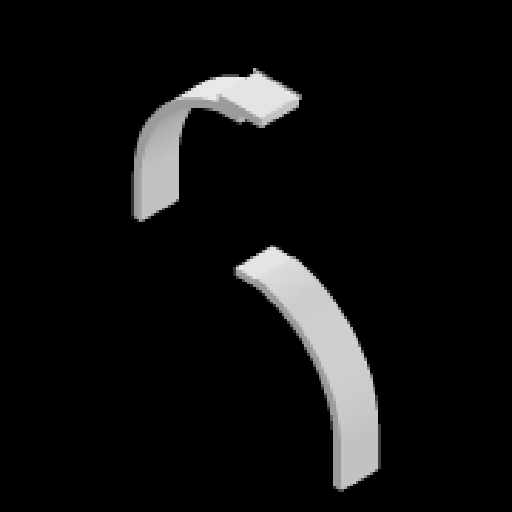
# Autodesk Inventor part: intakeConstraint
Saved by Autodesk Inventor 2024.1 (Build 281209000, 209)
## iProperties
Created: 2025-05-14
Part Number: intakeConstraint
Material: Generic
Document SubType Name: Modeling
Designer: Teddy
Density: 1 g/cm^3
Appearance: Default
Author: Teddy
Autodesk Inventor part; units mm, degrees
ref_plane "YZ Plane" through (0, 0, 0) normal (1, 0, 0) x (0, 1, 0)
ref_plane "XZ Plane" through (0, 0, 0) normal (0, 1, 0) x (-1, 0, 0)
ref_plane "XY Plane" through (0, 0, 0) normal (0, 0, 1) x (1, 0, 0)
ref_plane "Work Plane1" through (0, 0, 0) normal (0, 0, 1) x (1, 0, 0)
sketch "Sketch1" plane through (0, 0, 0) normal (0, 0, 1) x (1, 0, 0)
  line L0 (-103.1875, -92.8688) -> (-103.1875, -100.8761)
  line L1 (-2.3812, 0) -> (-35.7187, 0)
  line L2 (63.5, -115.8875) -> (63.5, -53.6292)
  line L3 (62.7062, -115.8875) -> (51.816, -115.8875)
  line L4 (-38.1, 13.2715) -> (-38.1, 2.3812)
  line L5 (0, 2.3812) -> (0, 13.2715)
  line L6 (63.5, -115.8875) -> (57.15, -115.8875)
  line L7 (57.15, -115.8875) -> (57.15, -86.36)
  line L8 (57.15, -86.36) -> (63.5, -86.36)
  line L9 (63.5, -86.36) -> (63.5, -115.8875)
  line L10 (-101.6, -115.8875) -> (-95.25, -115.8875)
  line L11 (-95.25, -115.8875) -> (-95.25, -86.36)
  line L12 (-95.25, -86.36) -> (-101.6, -86.36)
  line L13 (-101.6, -86.36) -> (-101.6, -115.8875)
  arc A0 (63.5, -86.36) -> (-101.6, -86.36) centre (-19.05, -86.36) ccw
  arc A1 (57.15, -86.36) -> (-95.25, -86.36) centre (-19.05, -86.36) ccw
  line L14 (-101.6, -104.2768) -> (-101.6, -115.8875)
  line L15 (-35.7187, 0) -> (-35.7187, -5.5104)
  line L16 (-2.3812, 0) -> (-2.3812, -5.5104)
  line L17 (-35.7187, 0) -> (-2.3812, 0)
  line L18 (-35.7187, -12.0055) -> (-2.3812, -12.0055)
  line L19 (-19.05, -12.0055) -> (-19.05, -6.6462)
  line L20 (-19.05, -6.6462) -> (-2.3812, -6.6462)
  line L21 (-2.3812, -6.6462) -> (-2.3812, -5.5104)
  point P0 (0, 0)
  point P1 (57.2611, -115.8875)
  point P2 (-19.05, 0)
  point P3 (-19.05, -3.81)
extrude "Extrusion1" add sketch "Sketch1" along normal blind 29.21 contours L16 A0 L15 L1 | L21 L20 L19 A1 L12 A0 | L12 L11 L10 L13 | L19 L18 A1 picked at (-28.3271, -11.6643)
sketch "Sketch2" plane through (0, 0, 29.21) normal (0, 0, 1) x (1, 0, 0)
  line L0 (-77.5465, -167.288) -> (-77.5465, -175.2953)
  line L1 (23.2597, -74.4192) -> (-10.0778, -74.4192)
  line L2 (89.141, -190.3067) -> (89.141, -128.0485)
  line L3 (88.3472, -190.3067) -> (77.457, -190.3067)
  line L4 (-12.459, -61.1477) -> (-12.459, -72.038)
  line L5 (25.641, -72.038) -> (25.641, -61.1477)
  line L6 (89.141, -190.3067) -> (82.791, -190.3067)
  line L7 (82.791, -190.3067) -> (82.791, -160.7792)
  line L8 (82.791, -160.7792) -> (89.141, -160.7792)
  line L9 (89.141, -160.7792) -> (89.141, -190.3067)
  line L10 (-75.959, -190.3067) -> (-69.609, -190.3067)
  line L11 (-69.609, -190.3067) -> (-69.609, -160.7792)
  line L12 (-69.609, -160.7792) -> (-75.959, -160.7792)
  line L13 (-75.959, -160.7792) -> (-75.959, -190.3067)
  arc A0 (89.141, -160.7792) -> (-75.959, -160.7792) centre (6.591, -160.7792) ccw
  arc A1 (82.791, -160.7792) -> (-69.609, -160.7792) centre (6.591, -160.7792) ccw
  line L14 (-75.959, -178.6961) -> (-75.959, -190.3067)
  line L15 (-10.0778, -74.4192) -> (-10.0778, -79.9296)
  line L16 (23.2597, -74.4192) -> (23.2597, -79.9296)
  line L17 (-10.0778, -74.4192) -> (23.2597, -74.4192)
  line L18 (-10.0778, -86.4247) -> (23.2597, -86.4247)
  line L19 (6.591, -86.4247) -> (6.591, -81.0655)
  line L20 (6.591, -81.0655) -> (23.2597, -81.0655)
  line L21 (23.2597, -81.0655) -> (23.2597, -79.9296)
  point P0 (0, 0)
  point P1 (25.641, -74.4192)
  point P2 (82.9021, -190.3067)
  point P3 (6.591, -74.4192)
  point P4 (6.591, -78.2292)
  dimension "d7" = 6.35
  dimension "d8" = 6.35
  dimension "d9" = 3.81
  constraints: 44 end point, 9 point on circle, 6 equal length, 5 tangent, 4 perpendicular, 3 midpoint, 2 centre point, 2 horizontal, 2 horizontal alignment, 2 point on line, 2 vertical, 1 coincident
  measures "d7" distance of L7.end L8.end
  measures "d8" distance of L12.end L11.end
  measures "d9" distance of point (6.591, -74.419) point (6.591, -78.229)
extrude "Extrusion2" add sketch "Sketch2" along normal blind 29.21 separate body contours A0 L8 A1 L19 L20 L21 | L2 L6 L3 L7 L8 | L18 L19 A1 picked at (15.8681, -86.0836)
sketch "Sketch3" plane through (-95.25, -115.8875, 0) normal (1, 0, 0) x (0, 0, -1)
  circle A0 centre (-8.255, 6.35) radius 2.286
  circle A1 centre (-20.955, 6.35) radius 2.286
  line L0 (0, 0) -> (0, 29.5275) projected
  line L1 (0, 0) -> (-29.21, 0) projected
  point P0 (0, 115.8875)
  dimension "d12" = 4.572
  dimension "d13" = 4.572
  dimension "d14" = 12.7
  dimension "d15" = 8.255
  dimension "d42" = 6.35
  constraints: 2 centre point, 1 horizontal alignment
  measures "d12" diameter of A0
  measures "d13" diameter of A1
  measures "d14" distance of A0.centre A1.centre
  measures "d15" distance from line of L0 A0.centre
  measures "d42" distance from line of L1 A0.centre
extrude "Extrusion3" cut sketch "Sketch3" against normal blind 29.21 bodies 1
sketch "Sketch4" plane through (-35.7187, -12.0055, 0) normal (0, -1, 0) x (1, 0, 0)
  circle A0 centre (10.3187, 20.955) radius 2.286
  circle A1 centre (10.3187, 8.255) radius 2.286
  circle A2 centre (23.0187, 20.955) radius 2.286
  circle A3 centre (23.0187, 8.255) radius 2.286
  line L0 (16.6688, 0) -> (16.6687, 29.21) projected
  line L1 (0, 0) -> (16.6688, 0) projected
  point P0 (35.7187, 0)
  dimension "d18" = 4.572
  dimension "d19" = 4.572
  dimension "d20" = 12.7
  dimension "d21" = 4.572
  dimension "d22" = 4.572
  dimension "d23" = 12.7
  dimension "d24" = 6.35
  dimension "d25" = 8.255
  constraints: 4 centre point, 2 horizontal alignment, 2 vertical alignment
  measures "d18" diameter of A0
  measures "d19" diameter of A1
  measures "d20" distance of A1.centre A0.centre
  measures "d21" diameter of A2
  measures "d22" diameter of A3
  measures "d23" distance of A3.centre A1.centre
  measures "d24" distance from line of L0 A3.centre
  measures "d25" distance from line of L1 A1.centre
extrude "Extrusion4" cut sketch "Sketch4" against normal blind 29.21 bodies 1
sketch "Sketch5" plane through (6.591, -81.0655, 29.21) normal (0, 1, 0) x (1, 0, 0)
  circle A0 centre (6.35, -20.955) radius 2.286
  circle A1 centre (6.35, -8.255) radius 2.286
  line L0 (16.6688, -29.21) -> (0, -29.21) projected
  line L1 (0, 0) -> (0, -29.21) projected
  point P0 (-6.591, 29.21)
  dimension "d28" = 4.572
  dimension "d29" = 4.572
  dimension "d30" = 12.7
  dimension "d31" = 8.255
  dimension "d32" = 6.35
  constraints: 2 centre point, 1 vertical alignment
  measures "d28" diameter of A0
  measures "d29" diameter of A1
  measures "d30" distance of A0.centre A1.centre
  measures "d31" distance from line of L0 A0.centre
  measures "d32" distance from line of L1 A0.centre
extrude "Extrusion5" cut sketch "Sketch5" against normal blind 29.21 bodies 2
sketch "Sketch6" plane through (82.791, -190.3067, 29.21) normal (-1, 0, 0) x (0, 0, 1)
  circle A0 centre (8.255, 6.35) radius 2.286
  circle A1 centre (20.955, 6.35) radius 2.286
  line L0 (0, 29.5275) -> (0, 0) projected
  line L1 (0, 0) -> (29.21, 0) projected
  point P0 (-29.21, 190.3067)
  dimension "d35" = 4.572
  dimension "d36" = 4.572
  dimension "d37" = 12.7
  dimension "d38" = 8.255
  dimension "d39" = 6.35
  constraints: 2 centre point, 1 horizontal alignment
  measures "d35" diameter of A0
  measures "d36" diameter of A1
  measures "d37" distance of A0.centre A1.centre
  measures "d38" distance from line of L0 A0.centre
  measures "d39" distance from line of L1 A1.centre
extrude "Extrusion6" cut sketch "Sketch6" against normal blind 29.21 bodies 2
body "Solid1"
body "Solid2"
